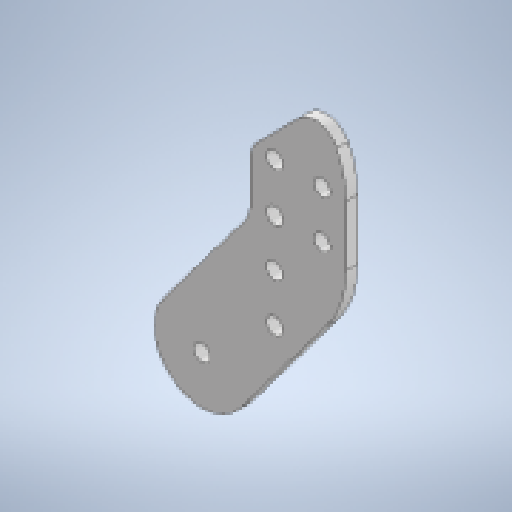
# Autodesk Inventor part: IntakeAftArm
Saved by Autodesk Inventor 2023 (Build 270158000, 158)
## iProperties
Created: 2022-11-09
Part Number: IntakeAftArm
Material: Generic
Document SubType Name: Modeling
Designer: Zac Hah
Density: 1 g/cm^3
Appearance: Default
Author: Zac Hah
Autodesk Inventor part; units mm, degrees
ref_plane "YZ Plane" through (0, 0, 0) normal (1, 0, 0) x (0, 1, 0)
ref_plane "XZ Plane" through (0, 0, 0) normal (0, 1, 0) x (-1, 0, 0)
ref_plane "XY Plane" through (0, 0, 0) normal (0, 0, 1) x (1, 0, 0)
sketch "Sketch1" plane through (0, 0, 0) normal (0, 0, 1) x (1, 0, 0)
  circle A0 centre (0, 0) radius 2.159
  circle A1 centre (0, 0) radius 12.7
  line L0 (0, 0) -> (0, 38.1) construction
  line L1 (0, 38.1) -> (12.827, 38.1) construction
  line L2 (12.827, 38.1) -> (12.827, 53.975)
  line L3 (12.827, 53.975) -> (30.7875, 71.9355)
  line L4 (12.827, 53.975) -> (38.227, 53.975) construction
  arc A2 (38.227, 53.975) -> (30.7875, 71.9355) centre (12.827, 53.975) ccw
  line L5 (12.827, 38.1) -> (-10.1397, 7.647)
  arc A3 (33.1064, 22.806) -> (38.227, 38.1) centre (12.827, 38.1) ccw
  line L6 (33.1064, 22.806) -> (10.1397, -7.647)
  line L7 (38.227, 38.1) -> (38.227, 53.975)
  circle A4 centre (31.877, 53.975) radius 2.159
  circle A5 centre (19.177, 53.975) radius 2.159
  circle A6 centre (31.877, 41.275) radius 2.159
  circle A7 centre (19.177, 41.275) radius 2.159
  circle A8 centre (31.877, 53.975) radius 6.35 construction
  circle A9 centre (19.177, 53.975) radius 6.35 construction
  circle A10 centre (19.177, 28.575) radius 2.159
  circle A11 centre (19.177, 15.875) radius 2.159
  dimension "d0" = 4.318
  dimension "d1" = 25.4
  dimension "d2" = 38.1
  dimension "d3" = 12.827
  dimension "d4" = 15.875
  dimension "d5" = 25.4
  dimension "d6" = 45
  dimension "d7" = 4.318
  dimension "d10" = 12.7
  dimension "d13" = 12.7
  dimension "d17" = 12.7
  dimension "d18" = 12.7
  constraints: 16 end point, 11 centre point, 6 coincident, 6 point on circle, 4 tangent, 4 vertical, 3 equal radius, 3 horizontal, 2 vertical alignment, 1 equal length, 1 horizontal alignment, 1 point on line, 9 other
  measures "d0" diameter of A0
  measures "d1" diameter of A1
  measures "d2" distance of L0.start L0.end
  measures "d3" distance of L0.end L1.end
  measures "d4" distance of L1.end L2.end
  measures "d5" distance of L2.end L3.end
  measures "d6" angle of L4 L3
  measures "d7" diameter of A4
  measures "d10" distance of A4.centre A5.centre
  measures "d13" distance of A4.centre A6.centre
  measures "d17" distance of A10.centre A7.centre
  measures "d18" distance of A11.centre A10.centre
extrude "Extrusion1" add sketch "Sketch1" along normal blind 3
fillet "Fillet1" radius 6.35 3 edges at (30.7875, 71.9355, 1.5) (12.827, 53.975, 1.5) (12.827, 38.1, 1.5)
body "Solid1"
